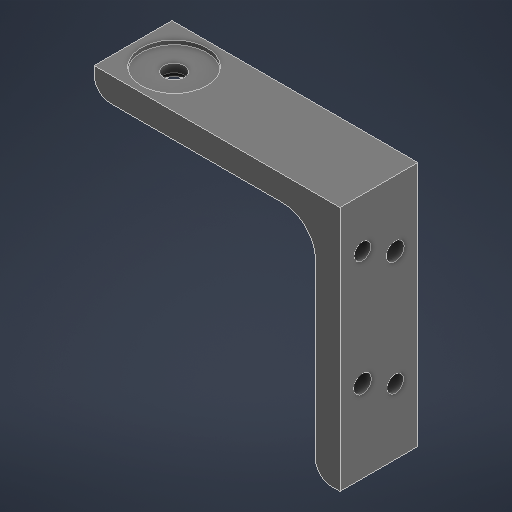
# Autodesk Inventor part: Kengyel3
Saved by Autodesk Inventor 2025 (Build 290162010, 162A)
## iProperties
Created: 2025-01-17
Part Number: Kengyel3
Material: Stainless Steel
Document SubType Name: Modeling
Designer: Tanár
Density: 8 g/cm^3
Appearance: Gray
Author: Tanár
Autodesk Inventor part; units mm, degrees
ref_plane "YZ Plane" through (0, 0, 0) normal (1, 0, 0) x (0, 1, 0)
ref_plane "XZ Plane" through (0, 0, 0) normal (0, 1, 0) x (-1, 0, 0)
ref_plane "XY Plane" through (0, 0, 0) normal (0, 0, 1) x (1, 0, 0)
sketch "Sketch1" plane through (0, 0, 0) normal (0, 0, 1) x (1, 0, 0)
  line L0 (0, -60) -> (0, 0)
  line L1 (0, 0) -> (-60, 0)
  line L2 (-60, 0) -> (-60, -2)
  line L3 (-56, -6) -> (-14, -6)
  line L4 (-6, -14) -> (-6, -56)
  line L5 (-2, -60) -> (0, -60)
  arc A0 (-6, -14) -> (-14, -6) centre (-14, -14) ccw
  arc A1 (-60, -2) -> (-56, -6) centre (-56, -2) ccw
  arc A2 (-6, -56) -> (-2, -60) centre (-2, -56) ccw
  point P0 (-6, -60)
  dimension "d0" = 60
  dimension "d1" = 6
  dimension "d2" = 8
  dimension "d3" = 4
  constraints: 12 end point, 7 perpendicular, 6 point on circle, 6 tangent, 3 centre point, 2 point on line, 1 coincident, 1 equal radius, 1 vertical
  measures "d0" distance of L0.start L0.end
  measures "d1" distance of point (-6, -60) L0.start
  measures "d2" radius of A0
  measures "d3" radius of A1
extrude "Extrusion1" add sketch "Sketch1" along normal mid plane 19
sketch "Sketch2" plane through (0, -60, 9.5) normal (1, 0, 0) x (0, 0, -1)
  line L0 (19, 60) -> (0, 60) projected
  line L1 (0, 0) -> (0, 60) projected
  point P0 (9.5, 60)
  point P1 (5.5, 48)
  point P2 (13.5, 44)
  point P3 (13.5, 16)
  point P4 (5.5, 20)
  dimension "d8" = 13.5
  dimension "d9" = 5.5
  dimension "d55" = 12
  dimension "d56" = 4
  dimension "d57" = 24
  dimension "d58" = 32
  constraints: 2 vertical alignment
  measures "d8" distance from line of point (13.5, 16) L1
  measures "d9" distance from line of point (5.5, 20) L1
  measures "d55" distance from line of point (5.5, 48) L0
  measures "d56" vertical distance of point (13.5, 44) point (5.5, 48)
  measures "d57" vertical distance of point (5.5, 20) point (13.5, 44)
  measures "d58" vertical distance of point (13.5, 16) point (5.5, 48)
hole "Hole1" at (0, -12, 4) at (0, -44, -4) direction (-1, 0, 0) diameter 4 end through all
sketch "Sketch3" plane through (-6, -56, 9.5) normal (-1, 0, 0) x (0, 0, 1)
  point P0 (-9.5, 56)
  point P1 (-5.5, 44)
  point P2 (-13.5, 12)
  point P3 (-13.5, 40)
  point P4 (-5.5, 16)
sketch "Sketch4" plane through (-60, 0, 9.5) normal (0, 1, 0) x (1, 0, 0)
  line L0 (60, 19) -> (60, 0) projected
  point P0 (60, 9.5)
  point P1 (10, 9.5)
  point P2 (60, 9.5)
  dimension "d33" = 50
  constraints: 1 horizontal alignment, 1 midpoint
  measures "d33" distance from line of point (10, 9.5) L0
hole "Hole4" at (-50, 0, 0) direction (0, -1, 0) diameter 16 depth 1 start extended yes
sketch "Sketch5" plane through (-56, -6, 9.5) normal (0, -1, 0) x (1, 0, 0)
  circle A0 centre (6, -9.5) radius 8 projected
  point P0 (56, -9.5)
  constraints: 1 coincident
hole "Hole5" at (-50, -6, 0) direction (0, 1, 0) diameter 5 end through all countersink diameter 11 countersink angle 90
hole "Hole6" at (-6, -40, 4) at (-6, -16, -4) direction (1, 0, 0) diameter 4.3 end through all start extended yes counterbore diameter 7.4 counterbore depth 2.5
body "Solid1"
